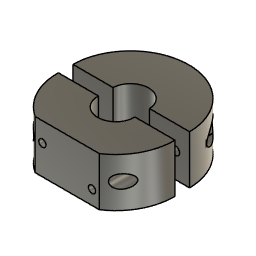
Mic stand clamp (Autodesk Fusion 360 design; units mm, degrees)
Autodesk Fusion 360 part; units mm, degrees
note: some values were not read from the file. Chosen so that the rebuilt part matches the saved one: which bodies a step acts on. Set by a fixed rule: which sketch regions a step uses.
sketch "Sketch1" plane through (0, 0, 0) normal (0, 0, 1) x (1, 0, 0)
  circle A0 centre (0, 0) radius 7.5
  circle A1 centre (0, 0) radius 24
  line L0 (-13.2023, -20.0425) -> (13.2023, -20.0425)
  line L1 (4.5796, 23.559) -> (-4.5, 23.559)
  dimension "d1" = 15
  dimension "d2" = 48
  constraint coincident A0.centre A1.centre
  constraint coincident A1 L0.start
  constraint coincident A1 L0.end
  constraint horizontal L0
  constraint coincident A1 L1.start
  constraint horizontal L1
  measures "d1" diameter of A0
  measures "d2" diameter of A1
extrude "Extrude1" add sketch "Sketch1" along normal blind 20 contours A1 L0 picked at (-0.1868, -15.8546) makes body 1
sketch "Sketch2" plane through (0, 0, 20) normal (0, 0, 1) x (-1, 0, 0)
  circle A0 centre (0, 0) radius 7.5
  line L0 (13.2023, 20.0425) -> (-13.2023, 20.0425)
  arc A1 (-13.2023, 20.0425) -> (13.2023, 20.0425) centre (0, 0) ccw
  line L1 (23.998, -0.3117) -> (-23.998, -0.3117)
  constraint coincident A1 L1.start
  constraint coincident A1 L1.end
  constraint horizontal L1
split "Split1" by curves path "Sketch2" along L1 bodies 1 makes body 2 at (-0.052, -15.8611, 0)
sketch "Sketch3" plane through (0, -20.0425, 0) normal (0, -1, 0) x (1, 0, 0)
  line L0 (-13.2023, 0) -> (13.2023, 0)
  line L1 (13.2023, 0) -> (13.2023, 20)
  line L2 (13.2023, 20) -> (-13.2023, 20)
  line L3 (-13.2023, 20) -> (-13.2023, 0)
  circle A0 centre (-18.2023, 10.3507) radius 1.7
  circle A1 centre (18.2023, 10.3507) radius 1.7
  dimension "d5" = 3.4
  dimension "d6" = 3.4
  dimension "d7" = 5
  dimension "d8" = 5
  measures "d5" diameter of A0
  measures "d6" diameter of A1
  measures "d7" distance of L3 A0.centre
  measures "d8" distance of L1 A1.centre
extrude "Extrude2" cut sketch "Sketch3" against normal blind 42 contours A0 | A1 bodies 1 2
sketch "Sketch4" plane through (0, -20.0425, 0) normal (0, -1, 0) x (1, 0, 0)
  line L0 (-13.2023, 0) -> (13.2023, 0)
  line L1 (13.2023, 0) -> (13.2023, 20)
  line L2 (13.2023, 20) -> (-13.2023, 20)
  line L3 (-13.2023, 20) -> (-13.2023, 0)
  circle A0 centre (-18.2023, 10.3508) radius 2.75
  circle A1 centre (18.1249, 10.3506) radius 2.75
  circle A2 centre (-18.2023, 10.3507) radius 1.7
  circle A3 centre (18.2023, 10.3507) radius 1.7
  dimension "d11" = 0.0001
  dimension "d12" = 5.5
  dimension "d13" = 0.0001
  dimension "d14" = 5.5
  measures "d11" distance of A0.centre A2.centre
  measures "d12" diameter of A0
  measures "d13" vertical distance of A1.centre A3.centre
  measures "d14" diameter of A1
extrude "Extrude3" cut sketch "Sketch4" against normal blind 14 contours A0 | A1 bodies 2
sketch "Sketch5" plane through (0, -20.0425, 0) normal (0, -1, 0) x (1, 0, 0)
  line L0 (-13.2023, 0) -> (13.2023, 0)
  line L1 (13.2023, 0) -> (13.2023, 20)
  line L2 (13.2023, 20) -> (-13.2023, 20)
  line L3 (-13.2023, 20) -> (-13.2023, 0)
  line L4 (19.9907, 13.4485) -> (16.1907, 13.4485)
  line L5 (16.1907, 13.4485) -> (14.2907, 10.1576)
  line L6 (14.2907, 10.1576) -> (16.1907, 6.8667)
  line L7 (19.9907, 6.8667) -> (16.1907, 6.8667)
  line L8 (19.9907, 6.8667) -> (21.8907, 10.1576)
  line L9 (21.8907, 10.1576) -> (19.9907, 13.4485)
  circle A0 centre (18.2023, 10.3507) radius 1.7
  dimension "d17" = 3.8
  dimension "d18" = 3.8
  dimension "d19" = 3.8
  dimension "d20" = 3.8
  dimension "d21" = 3.8
  dimension "d22" = 3.8
  dimension "d23" = 120
  dimension "d24" = 120
  dimension "d25" = 120
  dimension "d26" = 120
  dimension "d27" = 6.5818
  dimension "d28" = 3.291
  constraint horizontal L4
  constraint parallel L4 L7
  measures "d17" distance of L4.start L4.end
  measures "d18" distance of L4.end L5.end
  measures "d19" distance of L5.end L6.end
  measures "d20" distance of L6.end L7.start
  measures "d21" distance of L7.start L8.end
  measures "d22" distance of L4.start L8.end
  measures "d23" angle of L4 L5
  measures "d24" angle of L5 L6
  measures "d25" angle of L6 L7
  measures "d26" angle of L8 L9
  measures "d27" distance of L4 L7
  measures "d28" distance of L5 A0.centre
move_body "Move1" bodies 2 1 to x (1, 0, 0) y (0, 1, 0) z (0, 0, 1) at (0, -46, 0)
sketch "Sketch7" plane through (0, -20.0425, 0) normal (0, -1, 0) x (1, 0, 0)
  line L0 (-16.3808, 13.5057) -> (-20.1808, 13.5057)
  line L1 (-20.1808, 13.5057) -> (-22.0808, 10.2148)
  line L2 (-22.0808, 10.2148) -> (-20.1808, 6.9239)
  line L3 (-20.1808, 6.9239) -> (-16.3808, 6.9239)
  line L4 (-16.3808, 6.9239) -> (-14.4808, 10.2148)
  line L5 (-14.4808, 10.2148) -> (-16.3808, 13.5057)
  circle A0 centre (-18.2023, 10.3507) radius 1.7
  dimension "d30" = 3.8
  dimension "d31" = 3.8
  dimension "d32" = 3.8
  dimension "d33" = 3.8
  dimension "d34" = 3.8
  dimension "d35" = 120
  dimension "d36" = 120
  dimension "d37" = 120
  dimension "d38" = 6.5818
  dimension "d39" = 3.291
  dimension "d46" = 3.8
  constraint horizontal L0
  constraint parallel L0 L3
  constraint parallel L1 L4
  measures "d30" distance of L0.start L0.end
  measures "d31" distance of L0.end L1.end
  measures "d32" distance of L2.end L3.end
  measures "d33" distance of L1.end L2.end
  measures "d34" distance of L3.end L4.end
  measures "d35" angle of L0 L1
  measures "d36" angle of L1 L2
  measures "d37" angle of L2 L3
  measures "d38" distance of L0 L3
  measures "d39" distance of L1 A0.centre
  measures "d46" distance of L0.start L4.end
extrude "Extrude4" cut sketch "Sketch7" along normal blind 20 bodies 1
extrude "Extrude5" cut sketch "Sketch5" along normal blind 20 contours L4 L5 L6 L7 L8 L9 bodies 1
move_body "Move2" bodies 2 to x (1, 0, 0) y (0, 1, 0) z (0, 0, 1) at (0, -20, 0)
move_body "Move3" bodies 2 to x (1, 0, 0) y (0, 1, 0) z (0, 0, 1) at (0, 20, 0)
move_body "Move4" bodies 2 1 to x (1, 0, 0) y (0, 1, 0) z (0, 0, 1) at (0, 45, 0)
extrude "Extrude6" cut sketch "Sketch4" against normal blind 16 contours A0 | A1 bodies 2
move_body "Move5" bodies 1 to x (1, 0, 0) y (0, 1, 0) z (0, 0, 1) at (0, 11, 0)
move_body "Move6" bodies 1 to x (1, 0, 0) y (0, 1, 0) z (0, 0, 1) at (0, -11, 0)
move_body "Move7" bodies 1 to x (1, 0, 0) y (0, 1, 0) z (0, 0, 1) at (0, 14, 0)
sketch "Sketch8" plane through (0, -21.0425, 0) normal (0, -1, 0) x (1, 0, 0)
  line L0 (-13.2023, 0) -> (13.2023, 0)
  line L1 (13.2023, 0) -> (13.2023, 20)
  line L2 (13.2023, 20) -> (-13.2023, 20)
  line L3 (-13.2023, 20) -> (-13.2023, 0)
  circle A0 centre (18.2023, 10.3507) radius 4
  circle A1 centre (-18.2023, 10.3507) radius 4
  circle A2 centre (18.2023, 10.3507) radius 1.7
  circle A3 centre (-18.2023, 10.3507) radius 1.7
  dimension "d47" = 8
  dimension "d48" = 8
  dimension "d49" = 0
  dimension "d50" = 0
  dimension "d51" = 0
  dimension "d52" = 0
  dimension "d53" = 0
  dimension "d54" = 0
  measures "d47" diameter of A0
  measures "d48" diameter of A1
  measures "d49" distance of A0.centre A2.centre
  measures "d50" vertical distance of A1.centre A3.centre
  measures "d51" distance of A1.centre A3.centre
  measures "d52" distance of A0.centre A2.centre
  measures "d53" distance of A0.centre A2.centre
  measures "d54" distance of A0.centre A2.centre
move_body "Move8" bodies 1 2 to x (1, 0, 0) y (0, 1, 0) z (0, 0, 1) at (0, -55, 0)
extrude "Extrude7" cut sketch "Sketch8" along normal blind 12 contours A0 | A1 bodies 1
sketch "Sketch9" plane through (0, -76.0425, 0) normal (0, -1, 0) x (1, 0, 0)
  line L0 (-13.2023, 0) -> (13.2023, 0)
  line L1 (13.2023, 0) -> (13.2023, 20)
  line L2 (13.2023, 20) -> (-13.2023, 20)
  line L3 (-13.2023, 20) -> (-13.2023, 0)
  circle A0 centre (10.2023, 5.7707) radius 1.5
  circle A1 centre (-10.2023, 12.009) radius 1.5
  line L4 (-10.2023, 12.009) -> (8.2732, 12.009)
  line L5 (-10.2023, 12.009) -> (13.7054, 4.6997)
  dimension "d57" = 343
  dimension "d58" = 25
  dimension "d59" = 3
  dimension "d60" = 3
  dimension "d61" = 3
  dimension "d62" = 3
  constraint perpendicular L3 L4
  constraint coincident A1.centre L4.start
  constraint coincident A0.centre L5
  measures "d58" distance of A1.centre L5.end
  measures "d59" diameter of A1
  measures "d60" diameter of A0
  measures "d61" distance of L1 A0.centre
  measures "d62" distance of L3 A1.centre
extrude "Extrude8" cut sketch "Sketch9" against normal blind 9 contours A0 L5 | A0 L5 | A1 L4 L5 | A1 L4 L5 bodies 2
move_body "Move9" bodies 2 to x (1, 0, 0) y (0, 1, 0) z (0, 0, 1) at (0, 14, 0)
move_body "Move10" bodies 1 to x (1, 0, 0) y (0, 1, 0) z (0, 0, 1) at (0, 6, 0)
equation "d28 = ( 6.582 / 2 ) * 1 mm"
equation "d39 = ( 6.582 / 2 ) * 1 mm"
equation "d52 = 1.000E-05 mm"
equation "d53 = 1.000E-05 mm"
equation "d54 = 1.000E-05 mm"
equation "d57 = 360 deg - 17 deg"
